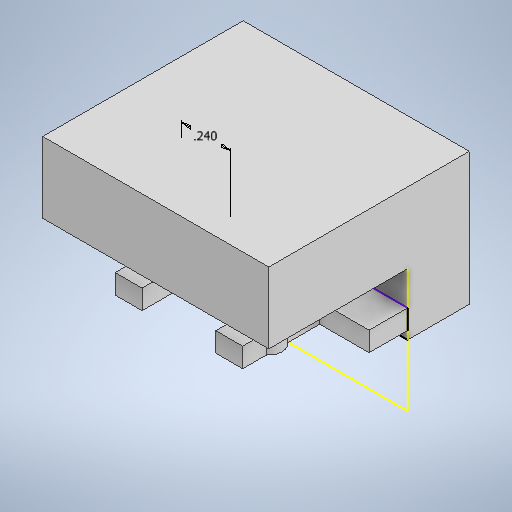
# Autodesk Inventor part: Attachment2
Saved by Autodesk Inventor 2025 (Build 290162010, 162A)
## iProperties
Created: 2026-02-26
Part Number: Attachment2
Material: Generic
Document SubType Name: Modeling
Designer: 925699
Density: 1 g/cm^3
Appearance: Default
Author: 925699
Autodesk Inventor part; units mm, degrees
ref_plane "YZ Plane" through (0, 0, 0) normal (1, 0, 0) x (0, 1, 0)
ref_plane "XZ Plane" through (0, 0, 0) normal (0, 1, 0) x (-1, 0, 0)
ref_plane "XY Plane" through (0, 0, 0) normal (0, 0, 1) x (1, 0, 0)
sketch "Sketch1" plane through (0, 0, 0) normal (0, 0, 1) x (1, 0, 0)
  line L0 (-6.3366, 6.9163) -> (21.6034, 6.9163)
  line L1 (21.6034, 6.9163) -> (21.6034, -8.3237)
  line L2 (21.6034, -8.3237) -> (-6.3366, -8.3237)
  line L3 (-6.3366, -8.3237) -> (-6.3366, 6.9163)
  point P0 (0, 0)
  dimension "d0" = 27.94
  dimension "d1" = 15.24
  constraints: 8 end point, 2 parallel, 1 horizontal, 1 perpendicular
  measures "d0" distance of L1.end L2.end
  measures "d1" distance of L0.end L1.end
extrude "Extrusion1" add sketch "Sketch1" along normal blind 7.62
sketch "Sketch2" plane through (0, 0, 7.62) normal (0, 0, 1) x (1, 0, 0)
  line L0 (-6.3366, 6.9163) -> (-6.3366, -8.3237) projected
  line L1 (21.6034, -8.3237) -> (21.6034, 6.9163) projected
  line L2 (21.6034, 0.3123) -> (21.6034, 2.7253)
  line L3 (-6.3366, 2.7253) -> (-6.3366, 0.3123)
  line L4 (21.6034, 6.9163) -> (-6.3366, 6.9163) projected
  line L5 (-6.3366, -8.3237) -> (21.6034, -8.3237) projected
  line L6 (0.9631, 2.7253) -> (-0.2406, 2.7253)
  line L7 (-0.2406, 0.3123) -> (0.9631, 0.3123)
  line L8 (-0.2406, 0.3123) -> (-0.2406, 2.7253)
  line L9 (-0.2406, 0.3123) -> (3.0821, 0.3123)
  line L10 (3.0821, 0.3123) -> (3.0821, 2.7253)
  line L11 (3.0821, 2.7253) -> (-0.2406, 2.7253)
  line L12 (-0.2406, 2.7253) -> (-0.2406, 0.3123)
  line L13 (14.3038, 2.7253) -> (15.5074, 2.7253)
  line L14 (15.5074, 0.3123) -> (14.3038, 0.3123)
  line L15 (15.5074, 0.3123) -> (15.5074, 2.7253)
  line L16 (15.5074, 0.3123) -> (12.1847, 0.3123)
  line L17 (12.1847, 0.3123) -> (12.1847, 2.7253)
  line L18 (12.1847, 2.7253) -> (15.5074, 2.7253)
  line L19 (15.5074, 2.7253) -> (15.5074, 0.3123)
  line L20 (-6.3366, -0.7037) -> (21.6034, -0.7037)
  line L21 (-6.3366, 2.7253) -> (21.6034, 2.7253)
  line L22 (21.6034, 2.7253) -> (21.6034, 0.3123)
  line L23 (21.6034, 0.3123) -> (-6.3366, 0.3123)
  line L24 (-6.3366, 0.3123) -> (-6.3366, 2.7253)
  point P0 (0, 0)
  point P1 (-0.2406, 1.5188)
  point P2 (15.2669, 0)
  point P3 (15.5074, 1.5188)
  dimension "d6" = 6.096
  constraints: 42 end point, 6 parallel, 4 perpendicular, 3 horizontal, 3 midpoint, 2 point on line
  measures "d6" distance from line of point (-0.241, 1.519) L0
extrude "Extrusion2" add sketch "Sketch2" along normal blind 8.7376 contours L6 L11 L10 L9 L7 L8 | L15 L14 L16 L17 L18 L13
sketch "Sketch3" plane through (-0.2406, 2.7253, 7.62) normal (0, 1, 0) x (1, 0, 0)
  line L0 (3.3227, -8.7376) -> (0, -8.7376) projected
  line L1 (3.3227, -11.3552) -> (0, -11.3552)
  line L2 (0, -11.3552) -> (0, -8.7376)
  line L3 (3.3227, -8.7376) -> (0, -8.7376)
  line L4 (-6.096, 7.62) -> (21.844, 7.62) projected
  line L5 (3.3227, -11.3552) -> (3.3227, -8.7376)
  arc A0 (0, -8.7376) -> (0, -11.3552) centre (1.0363, -10.0464) ccw
  line L6 (12.4253, -8.7376) -> (15.748, -8.7376)
  line L7 (12.4253, -11.3552) -> (15.748, -11.3552)
  line L8 (15.748, -11.3552) -> (15.748, -8.7376)
  line L9 (12.4253, -8.7376) -> (15.748, -8.7376)
  line L10 (12.4253, -11.3552) -> (12.4253, -8.7376)
  arc A1 (15.748, -11.3552) -> (15.748, -8.7376) centre (14.7117, -10.0464) ccw
  point P0 (0.2406, 7.62)
  constraints: 18 end point, 4 point on circle, 2 centre point, 1 collinear, 1 horizontal, 1 perpendicular, 1 vertical
extrude "Extrusion3" add sketch "Sketch3" against normal up to surface (2.413 mm away)
extrude "Extrusion4" add sketch "Sketch2" along normal blind 14.2875 contours L6 L11 L10 L9 L7 L8 | L15 L14 L16 L17 L18 L13
sketch "Sketch4" plane through (-6.3366, 6.9163, 0) normal (0, 1, 0) x (1, 0, 0)
  point P0 (6.3366, 0)
sketch "Sketch5" plane through (0, 0, 7.62) normal (0, 0, 1) x (1, 0, 0)
  line L0 (21.6034, 6.9163) -> (-6.3366, 6.9163) projected
  line L1 (-6.3366, 15.6735) -> (21.6034, 15.6735)
  line L2 (21.6034, 15.6735) -> (21.6034, 6.9163)
  line L3 (21.6034, 6.9163) -> (-6.3366, 6.9163)
  line L4 (-6.3366, 6.9163) -> (-6.3366, 15.6735)
  point P0 (0, 0)
  constraints: 8 end point, 2 parallel, 1 horizontal, 1 perpendicular
extrude "Extrusion5" add sketch "Sketch5" along normal blind 17.145 and the other way blind 7.62
extrude "Extrusion6" cut sketch "Sketch2" against normal blind 25.4 contours L20 L1 L5 L0
extrude "Extrusion7" add sketch "Sketch2" along normal blind 4.7625 contours L21 L8 L23 L0 | L1 L23 L15 L21 | L21 L17 L23 L10
body "Solid1"
